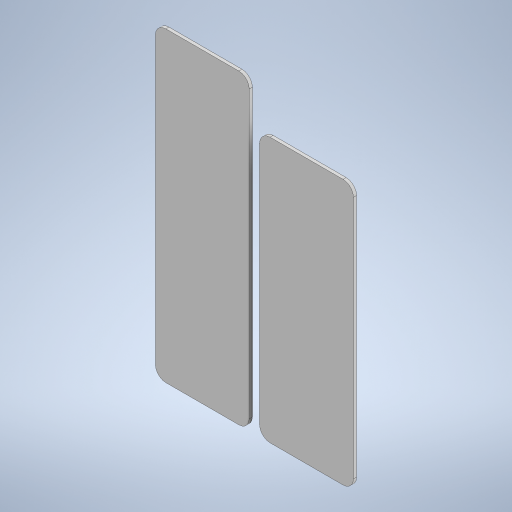
# Autodesk Inventor part: base 2 plate
Saved by Autodesk Inventor 2023.5 (Build 275446020, 446B)
## iProperties
Created: 2025-04-23
Part Number: base 2 plate
Material: Generic
Document SubType Name: Modeling
Designer: Lucky Sah
Density: 1 g/cm^3
Appearance: Default
Author: Lucky Sah
Autodesk Inventor part; units mm, degrees
ref_plane "YZ Plane" through (0, 0, 0) normal (1, 0, 0) x (0, 1, 0)
ref_plane "XZ Plane" through (0, 0, 0) normal (0, 1, 0) x (-1, 0, 0)
ref_plane "XY Plane" through (0, 0, 0) normal (0, 0, 1) x (1, 0, 0)
sketch "Sketch1" plane through (0, 0, 0) normal (0, 0, 1) x (1, 0, 0)
  line L0 (-175.0131, 86.2523) -> (-215.0131, 86.2523)
  line L1 (-225.0131, 76.2523) -> (-225.0131, -50.7477)
  line L2 (-215.0131, -60.7477) -> (-175.0131, -60.7477)
  line L3 (-230.0131, 57.2523) -> (-230.0131, -50.7477)
  arc A0 (-215.0131, 86.2523) -> (-225.0131, 76.2523) centre (-215.0131, 76.2523) ccw
  arc A1 (-225.0131, -50.7477) -> (-215.0131, -60.7477) centre (-215.0131, -50.7477) ccw
  arc A2 (-240.0131, -60.7477) -> (-230.0131, -50.7477) centre (-240.0131, -50.7477) ccw
  arc A3 (-230.0131, 57.2523) -> (-240.0131, 67.2523) centre (-240.0131, 57.2523) ccw
  line L4 (-210.0131, 86.2523) -> (-210.0131, -60.7477)
  circle A4 centre (-210.0131, 12.7523) radius 1.75
  circle A5 centre (-210.0131, -40.7477) radius 1.75
  circle A6 centre (-210.0131, 66.2523) radius 1.75
  line L5 (-235.0131, 86.2523) -> (-270.0131, 86.2523)
  line L6 (-275.0131, 81.2523) -> (-275.0131, -55.7477)
  line L7 (-270.0131, -60.7477) -> (-235.0131, -60.7477)
  line L8 (-230.0131, -55.7477) -> (-230.0131, 81.2523)
  line L9 (-220.0131, 66.2523) -> (-185.0131, 66.2523)
  line L10 (-180.0131, 61.2523) -> (-180.0131, -55.7477)
  line L11 (-185.0131, -60.7477) -> (-220.0131, -60.7477)
  line L12 (-225.0131, -55.7477) -> (-225.0131, 61.2523)
  arc A7 (-180.0131, 61.2523) -> (-185.0131, 66.2523) centre (-185.0131, 61.2523) ccw
  arc A8 (-220.0131, 66.2523) -> (-225.0131, 61.2523) centre (-220.0131, 61.2523) ccw
  arc A9 (-225.0131, -55.7477) -> (-220.0131, -60.7477) centre (-220.0131, -55.7477) ccw
  arc A10 (-185.0131, -60.7477) -> (-180.0131, -55.7477) centre (-185.0131, -55.7477) ccw
  arc A11 (-235.0131, -60.7477) -> (-230.0131, -55.7477) centre (-235.0131, -55.7477) ccw
  arc A12 (-275.0131, -55.7477) -> (-270.0131, -60.7477) centre (-270.0131, -55.7477) ccw
  arc A13 (-270.0131, 86.2523) -> (-275.0131, 81.2523) centre (-270.0131, 81.2523) ccw
  arc A14 (-230.0131, 81.2523) -> (-235.0131, 86.2523) centre (-235.0131, 81.2523) ccw
  point P0 (-225.0131, -60.7477)
  point P1 (-230.0131, -60.7477)
  point P2 (88.9869, -60.7477)
  point P3 (-171.0131, -60.7477)
  point P4 (88.9869, -60.7477)
  point P5 (92.9869, -60.7477)
  point P6 (-171.0131, -60.7477)
  point P7 (92.9869, -60.7477)
  point P8 (88.9869, -60.7477)
  point P9 (-275.0131, -60.7477)
  point P10 (-230.0131, -60.7477)
  point P11 (-180.0131, -60.7477)
  point P12 (-225.0131, -60.7477)
  dimension "d24" = 10
  dimension "d25" = -5
  dimension "d26" = 15
  dimension "d30" = 3.5
  dimension "d32" = 3.5
  dimension "d46" = 45
  dimension "d47" = 45
  dimension "d48" = 5
  dimension "d49" = 5
  dimension "d50" = 5
  dimension "d51" = 5
  dimension "d52" = 3.5
  dimension "d60" = 5
  constraints: 26 end point, 24 point on circle, 22 tangent, 17 point on line, 15 centre point, 9 equal radius, 5 parallel, 4 perpendicular, 3 horizontal, 1 midpoint
  measures "d24" radius of A0
  measures "d25" distance between parallel lines of L3 L1
  measures "d26" distance between parallel lines of L4 L1
  measures "d30" diameter of A4
  measures "d32" diameter of A5
  measures "d46" distance of point (-230.013, -60.748) point (-275.013, -60.748)
  measures "d47" distance of point (-180.013, -60.748) point (-225.013, -60.748)
  measures "d48" radius of A7
  measures "d49" radius of A8
  measures "d50" distance between parallel lines of L8 L1
  measures "d51" distance between parallel lines of L12 L3
  measures "d52" diameter of A6
  measures "d60" distance between parallel lines of L8 L12
extrude "Extrusion1" add sketch "Sketch1" along normal blind 1.5 contours L9 A6 L4 | L4 A6 L9 | L9 A7 L10 A10 L2 L4 A5 A4 A6 | A6 L4 A4 A5 L2 A1 L1 A8 L9 | A1 L11 A9 L12 | A4 L4 | L4 A4 | A5 L4 | L4 A5 | L3 A2 L7 A12 L6 A13 L5 A14 L8 | L8 A11 L7 A2 picked at (-209.6302, 65.158) picked at (-211.1651, 66.1225)
body "Solid1"
